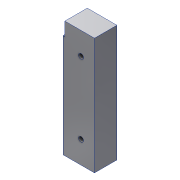
# Autodesk Inventor part: Distanzblock
Saved by Autodesk Inventor 2016 (Build 200138000, 138)
## iProperties
Created: 2015-07-27
Part Number: Distanzblock
Material: Aluminum 6061
Document SubType Name: Modeling
Density: 2.7 g/cm^3
Appearance: Aluminum - Flat
Autodesk Inventor part; units mm, degrees
ref_plane "YZ Plane" through (0, 0, 0) normal (1, 0, 0) x (0, 1, 0)
ref_plane "XZ Plane" through (0, 0, 0) normal (0, 1, 0) x (-1, 0, 0)
ref_plane "XY Plane" through (0, 0, 0) normal (0, 0, 1) x (1, 0, 0)
sketch "Sketch1" plane through (0, 0, 0) normal (0, 0, 1) x (1, 0, 0)
  line L0 (-17.5, -12.5) -> (17.5, -12.5)
  line L1 (17.5, -12.5) -> (17.5, 12.5)
  line L2 (17.5, 12.5) -> (-17.5, 12.5)
  line L3 (-17.5, 12.5) -> (-17.5, -12.5)
  line L4 (-17.5, -12.5) -> (17.5, 12.5) construction
  line L5 (17.5, -12.5) -> (-17.5, 12.5) construction
  point P0 (0, 0)
  dimension "d0" = 35
  dimension "d1" = 25
  constraints: 12 end point, 2 midpoint, 2 parallel, 1 horizontal, 1 perpendicular
  measures "d0" distance of L2.end L1.end
  measures "d1" distance of L1.end L0.end
extrude "Extrusion1" add sketch "Sketch1" along normal blind 130
sketch "Sketch2" plane through (-17.5, -12.5, 0) normal (0, -1, 0) x (1, 0, 0)
  line L0 (2, 115) -> (0, 115)
  line L1 (0, 115) -> (0, 130)
  line L2 (0, 130) -> (2, 130)
  line L3 (2, 130) -> (2, 115)
  line L4 (0, 0) -> (0, 130) projected
  line L5 (0, 130) -> (35, 130) projected
  point P0 (17.5, 0)
  dimension "d4" = 2
  dimension "d5" = 15
  constraints: 8 end point, 2 collinear, 2 parallel, 1 horizontal, 1 perpendicular
  measures "d4" distance of L0.start L0.end
  measures "d5" distance of L2.end L0.start
extrude "Extrusion2" cut sketch "Sketch2" against normal through all
sketch "Sketch3" plane through (-17.5, 12.5, 0) normal (0, 1, 0) x (1, 0, 0)
  line L0 (35, 0) -> (0, 0) projected
  line L1 (35, -130) -> (2, -130) projected
  line L2 (35, 0) -> (35, -130) projected
  point P0 (17.5, 0)
  point P1 (20, -25)
  point P2 (20, -105)
  dimension "d18" = 25
  dimension "d19" = 25
  dimension "d20" = 15
  constraints: 1 vertical alignment
  measures "d18" distance from line of point (20, -25) L0
  measures "d19" distance from line of L1 point (20, -105)
  measures "d20" distance from line of point (20, -25) L2
hole "Hole1" at (2.5, 12.5, 25) at (2.5, 12.5, 105) direction (0, -1, 0) diameter 5.5 end through all counterbore diameter 10 counterbore depth 9 clearance for "Socket Head Cap Screw ISO 4762" size "M5" standard "ISO"
equation "\"d19\" = d18"
body "Solid1"
